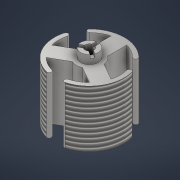
# Autodesk Inventor part: Suporte Bobinas
Saved by Autodesk Inventor 2021 (Build 250183000, 183)
## iProperties
Created: 2021-01-22
Part Number: Suporte Bobinas
Material: Genérico
Document SubType Name: Modeling
Designer: João
Density: 1 g/cm^3
Appearance: Padrão
Author: João
Autodesk Inventor part; units mm, degrees
ref_plane "YZ Plane" through (0, 0, 0) normal (1, 0, 0) x (0, 1, 0)
ref_plane "XZ Plane" through (0, 0, 0) normal (0, 1, 0) x (-1, 0, 0)
ref_plane "XY Plane" through (0, 0, 0) normal (0, 0, 1) x (1, 0, 0)
sketch "Esboço1" plane through (0, 0, 0) normal (0, 1, 0) x (-1, 0, 0)
  circle A0 centre (0, 0) radius 0.5
  circle A1 centre (0, 0) radius 1
  circle A2 centre (0, 0) radius 1.5
  dimension "d0" = 1
  dimension "d1" = 2
  dimension "d2" = 3
  constraints: 3 centre point, 3 coincident
  measures "d0" diameter of A0
  measures "d1" diameter of A1
  measures "d2" diameter of A2
extrude "Extrusão1" add sketch "Esboço1" against normal blind 6.5 contours A1 | A2
sketch "Esboço3" plane through (0, 0, 0) normal (0, 1, 0) x (1, 0, 0)
  line L0 (0.9, 0) -> (-0.9, 0)
  line L1 (-0.9, 0) -> (-0.9, 4)
  line L2 (-0.9, 4) -> (0.9, 4)
  line L3 (0.9, 4) -> (0.9, 0)
  line L4 (-0.45, 0.7794) -> (0.45, -0.7794)
  line L5 (0.45, -0.7794) -> (-3.0141, -2.7794)
  line L6 (-3.0141, -2.7794) -> (-3.9141, -1.2206)
  line L7 (-3.9141, -1.2206) -> (-0.45, 0.7794)
  line L8 (-0.45, -0.7794) -> (0.45, 0.7794)
  line L9 (0.45, 0.7794) -> (3.9141, -1.2206)
  line L10 (3.9141, -1.2206) -> (3.0141, -2.7794)
  line L11 (3.0141, -2.7794) -> (-0.45, -0.7794)
  circle A0 centre (0, 0) radius 0.5 projected
  circle A1 centre (0, 0) radius 4
  circle A2 centre (0, 0) radius 3.5
  line L12 (0, 0) -> (4, 0) construction
  line L13 (0.375, -0.6495) -> (3.7777, 1.315)
  line L14 (-0.375, 0.6495) -> (3.0277, 2.614)
  line L15 (-0.375, -0.6495) -> (-3.7777, 1.315)
  line L16 (0.375, 0.6495) -> (-3.0277, 2.614)
  line L17 (0.75, 0) -> (0.75, -3.9291)
  line L18 (-0.75, 0) -> (-0.75, -3.9291)
  circle A3 centre (0, 0) radius 1.5 projected
  circle A4 centre (0, 0) radius 0.5 projected
  point P0 (0.9, 1.2)
  point P1 (0.9, 3.3823)
  point P2 (2.5857, 2.3589)
  point P3 (-2.5857, 2.3589)
  point P4 (-0.9, 3.3823)
  point P5 (-0.9, 1.2)
  point P6 (0.5892, -1.3794)
  point P7 (2.4792, -2.4706)
  point P8 (0.75, -3.4187)
  point P9 (3.3357, 1.0598)
  point P10 (3.3792, -0.9117)
  point P11 (1.4892, 0.1794)
  point P12 (-1.4892, 0.1794)
  point P13 (-3.3792, -0.9117)
  point P14 (-3.3357, 1.0598)
  point P15 (-0.75, -3.4187)
  point P16 (-2.4792, -2.4706)
  point P17 (-0.5892, -1.3794)
  dimension "d9" = 360
  dimension "d11" = 7
  dimension "d21" = 360
  constraints: 38 end point, 4 coincident, 2 centre point, 2 horizontal, 2 parallel, 2 point on circle, 2 point on line, 1 perpendicular, 45 other
  measures "d11" diameter of A2
extrude "Extrusão2" add sketch "Esboço3" against normal blind 6.5 contours A3 L14 L3 | L9 L13 A3 | L13 L9 A2 L11 L17 A3 | L17 L11 A3 | L14 A3 L16 L1 A2 L3 | A2 L1 A1 L3 | L3 A1 L14 A2 | A3 L1 L16 | A2 L13 A1 L9 | L9 A1 L11 A2 | L11 A1 L17 A2 | L5 L18 A3 | A2 L16 A1 L1 | L18 A1 L5 A2 | L5 A2 L7 L15 A3 L18 | A3 L15 L7 | L5 A1 L7 A2 | A2 L7 A1 L15
fillet "Arredondamento1" radius 0.25 12 edges at (3.0277, -3.25, -2.614) (0.75, -3.25, 3.9291) (0.75, -3.25, 3.4187) (-0.75, -3.25, 3.9291) (-0.75, -3.25, 3.4187) (-3.3357, -3.25, -1.0598) (-3.7777, -3.25, -1.315) (-2.5857, -3.25, -2.3589) (-3.0277, -3.25, -2.614) (3.7777, -3.25, -1.315) (3.3357, -3.25, -1.0598) (2.5857, -3.25, -2.3589)
sketch "Esboço4" plane through (0, 0, 0) normal (0, 1, 0) x (1, 0, 0)
  circle A0 centre (0, 0) radius 1
  circle A1 centre (0, 0) radius 0.5 projected
  dimension "d26" = 2
  constraints: 1 centre point, 1 coincident
  measures "d26" diameter of A0
extrude "Extrusão3" add sketch "Esboço4" along normal blind 1 and the other way blind 7.5
sketch "Esboço5" plane through (0, 1, 0) normal (0, 1, 0) x (1, 0, 0)
  circle A0 centre (0, 0) radius 1 projected
  circle A1 centre (0, 0) radius 0.5 projected
  line L0 (0.2, 0) -> (-0.2, 0)
  line L1 (-0.2, 0) -> (-0.2, 0.9798)
  line L2 (0.2, 0.9798) -> (0.2, 0)
  line L3 (-0.1, 0.1732) -> (0.1, -0.1732)
  line L4 (0.1, -0.1732) -> (-0.7485, -0.6631)
  line L5 (-0.9485, -0.3167) -> (-0.1, 0.1732)
  line L6 (-0.1, -0.1732) -> (0.1, 0.1732)
  line L7 (0.1, 0.1732) -> (0.9485, -0.3167)
  line L8 (0.7485, -0.6631) -> (-0.1, -0.1732)
  point P0 (0.2, 0.4583)
  point P1 (-0.2, 0.4583)
  point P2 (0.2969, -0.4023)
  point P3 (0.7485, -0.6631)
  point P4 (0.4969, -0.0559)
  point P5 (-0.4969, -0.0559)
  point P6 (-0.9485, -0.3167)
  point P7 (-0.7485, -0.6631)
  point P8 (-0.2969, -0.4023)
  dimension "d35" = 360
  dimension "d39" = 0.4
  dimension "d40" = 0.2
  constraints: 18 end point, 2 coincident, 2 point on circle, 1 parallel, 29 other
  measures "d39" distance between parallel lines of L1 L2
  measures "d40" distance from line of point (0, 0) L2
extrude "Extrusão4" cut sketch "Esboço5" against normal blind 0.4 contours L2 A1 L1 A0 | A0 L8 A1 L7 | L5 A1 L4 A0
sketch "Esboço6" plane through (0, -7.5, 0) normal (0, -1, 0) x (1, 0, 0)
  arc A0 (0.9485, 0.3167) -> (0.7485, 0.6631) centre (0, 0) ccw projected
  line L0 (0.4969, 0.0559) -> (0.9485, 0.3167) projected
  arc A1 (0.4969, 0.0559) -> (0.2969, 0.4023) centre (0, 0) ccw projected
  line L1 (0.7485, 0.6631) -> (0.2969, 0.4023) projected
  circle A2 centre (0, 0) radius 1 projected
  arc A3 (-0.7485, 0.6631) -> (-0.9485, 0.3167) centre (0, 0) ccw projected
  line L2 (-0.2969, 0.4023) -> (-0.7485, 0.6631) projected
  arc A4 (-0.2969, 0.4023) -> (-0.4969, 0.0559) centre (0, 0) ccw projected
  line L3 (-0.9485, 0.3167) -> (-0.4969, 0.0559) projected
  arc A5 (-0.2, -0.9798) -> (0.2, -0.9798) centre (0, 0) ccw projected
  line L4 (-0.2, -0.4583) -> (-0.2, -0.9798) projected
  arc A6 (-0.2, -0.4583) -> (0.2, -0.4583) centre (0, 0) ccw projected
  line L5 (0.2, -0.9798) -> (0.2, -0.4583) projected
  point P0 (-0.2, -0.9798)
  point P1 (0.2, -0.9798)
  point P2 (-0.7485, 0.6631)
  point P3 (-0.9485, 0.3167)
extrude "Extrusão5" cut sketch "Esboço6" against normal blind 0.4 contours L0 A1 L1 A0 | L2 A4 L3 A2 | A2 L4 A6 L5
thread "Rosca1" size "M8x0.5" class "6g" standard "ANSI Metric M Profile" length 6.5
